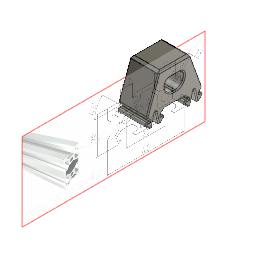
ENDER3_RUBBER_FEET_v2 (Autodesk Fusion 360 design; units mm, degrees)
Autodesk Fusion 360 part; units mm, degrees
sketch "Sketch1" plane through (0, 0, 0) normal (1, 0, 0) x (0, 1, 0)
  line L0 (20, 11.6667) -> (-20, 11.6667)
  line L1 (-20, 11.6667) -> (-20, -11.6667)
  line L2 (-20, -11.6667) -> (20, -11.6667)
  line L3 (20, -11.6667) -> (20, 11.6667)
  line L4 (20, 11.6667) -> (-20, -11.6667) construction
  line L5 (-20, 11.6667) -> (20, -11.6667) construction
  line L6 (-15.4, 8.6) -> (-15.4, 10.1)
  line L7 (-15.4, 10.1) -> (-13.2, 10.2)
  line L8 (-13.2, 10.2) -> (-13.2, 10.4)
  line L9 (-13.2, 10.4) -> (-14.6998, 11.8912)
  line L10 (-15.4, 8.6) -> (-12.8, 6.1)
  line L11 (-12.8, 6.1) -> (-7.2, 6.1)
  line L12 (-7.2, 6.1) -> (-4.6, 8.6)
  line L13 (-4.6, 8.6) -> (-4.6, 10)
  line L14 (-4.6, 10) -> (-6.9, 10)
  line L15 (-6.9, 10) -> (-6.9, 10.4)
  line L16 (-6.9, 10.4) -> (-5.2, 11.9)
  line L17 (-5.2, 11.9) -> (5.1942, 11.9)
  line L18 (5.1942, 11.9) -> (6.9277, 10.3512)
  line L19 (6.9277, 10.3512) -> (6.9277, 10.1)
  line L20 (6.9277, 10.1) -> (4.6, 10.1)
  line L21 (4.6, 10.1) -> (4.6, 8.6)
  line L22 (4.6, 8.6) -> (7.1681, 6.1554)
  line L23 (7.1681, 6.1554) -> (12.8, 6.1554)
  line L24 (12.8, 6.1554) -> (15.4, 8.6)
  line L25 (15.4, 8.6) -> (15.4, 10.1)
  line L26 (15.4, 10.1) -> (13.1, 10.1)
  line L27 (13.1, 10.1) -> (13.1, 10.4)
  line L28 (13.1, 10.4) -> (14.7, 11.9)
  line L29 (-12.95, 10.504) -> (-14.5235, 12.0685)
  line L30 (-12.95, 9.9611) -> (-12.95, 10.504)
  line L31 (-15.15, 9.8611) -> (-12.95, 9.9611)
  line L32 (-15.15, 8.7064) -> (-15.15, 9.8611)
  line L33 (-15.15, 8.7064) -> (-12.6993, 6.35)
  line L34 (-12.6993, 6.35) -> (-7.3007, 6.35)
  line L35 (-7.3007, 6.35) -> (-4.85, 8.7064)
  line L36 (-4.85, 8.7064) -> (-4.85, 9.75)
  line L37 (-4.85, 9.75) -> (-7.15, 9.75)
  line L38 (-7.15, 9.75) -> (-7.15, 10.5128)
  line L39 (-7.15, 10.5128) -> (-5.2945, 12.15)
  line L40 (-5.2945, 12.15) -> (5.2897, 12.15)
  line L41 (5.2897, 12.15) -> (7.1777, 10.4631)
  line L42 (7.1777, 10.4631) -> (7.1777, 9.85)
  line L43 (7.1777, 9.85) -> (4.85, 9.85)
  line L44 (4.85, 9.85) -> (4.85, 8.7072)
  line L45 (4.85, 8.7072) -> (7.268, 6.4054)
  line L46 (7.268, 6.4054) -> (12.7009, 6.4054)
  line L47 (12.7009, 6.4054) -> (15.15, 8.7081)
  line L48 (15.15, 8.7081) -> (15.15, 9.85)
  line L49 (15.15, 9.85) -> (12.85, 9.85)
  line L50 (12.85, 9.85) -> (12.85, 10.5083)
  line L51 (12.85, 10.5083) -> (14.529, 12.0824)
  line L52 (-0.0024, 12.15) -> (-0.0024, 30)
  line L53 (-0.0024, 30) -> (-8, 30)
  line L54 (-8, 30) -> (-14.5235, 12.0685)
  line L55 (-0.0024, 30) -> (7.9951, 30)
  line L56 (7.9951, 30) -> (14.5186, 12.0685)
  dimension "d1" = 40
  dimension "d2" = 0.25
  measures "d1" distance of L0.start L0.end
extrude "Extrude1" add sketch "Sketch1" along normal blind 15 contours L0 L41 L42 L43 L44 L45 L46 L47 L48 L49 L50 L51 | L0 L40 L41 L51 L52 L55 L56 | L0 L29 L39 L40 L52 L53 L54 | L0 L29 L30 L31 L32 L33 L34 L35 L36 L37 L38 L39
sketch "Sketch2" plane through (15, 0, 0) normal (1, 0, 0) x (0, 1, 0)
  line L0 (7.9951, 30) -> (-8, 30)
  line L1 (-8, 30) -> (-14.5235, 12.0685)
  line L2 (-14.5235, 12.0685) -> (-12.95, 10.504)
  line L3 (-12.95, 10.504) -> (-12.95, 9.9611)
  line L4 (-12.95, 9.9611) -> (-15.15, 9.8611)
  line L5 (-15.15, 9.8611) -> (-15.15, 8.7064)
  line L6 (-15.15, 8.7064) -> (-12.6993, 6.35)
  line L7 (-12.6993, 6.35) -> (-7.3007, 6.35)
  line L8 (-7.3007, 6.35) -> (-4.85, 8.7064)
  line L9 (-4.85, 8.7064) -> (-4.85, 9.75)
  line L10 (-4.85, 9.75) -> (-7.15, 9.75)
  line L11 (-7.15, 9.75) -> (-7.15, 10.5128)
  line L12 (-7.15, 10.5128) -> (-5.2945, 12.15)
  line L13 (-5.2945, 12.15) -> (5.2897, 12.15)
  line L14 (5.2897, 12.15) -> (7.1777, 10.4631)
  line L15 (7.1777, 10.4631) -> (7.1777, 9.85)
  line L16 (7.1777, 9.85) -> (4.85, 9.85)
  line L17 (4.85, 9.85) -> (4.85, 8.7072)
  line L18 (4.85, 8.7072) -> (7.268, 6.4054)
  line L19 (7.268, 6.4054) -> (12.7009, 6.4054)
  line L20 (12.7009, 6.4054) -> (15.15, 8.7081)
  line L21 (15.15, 8.7081) -> (15.15, 9.85)
  line L22 (15.15, 9.85) -> (12.85, 9.85)
  line L23 (12.85, 9.85) -> (12.85, 10.5083)
  line L24 (12.85, 10.5083) -> (14.5175, 12.0716)
  line L25 (14.5175, 12.0716) -> (7.9951, 30)
  line L26 (-10, 6.35) -> (-10, 13.85)
  line L27 (-10, 13.85) -> (-11.75, 6.35)
  line L28 (-11.75, 6.35) -> (-10, 6.35)
  line L29 (-0.0024, 30) -> (-0.0024, 12.15)
  line L30 (-10, 13.85) -> (-8.25, 6.35)
  line L31 (-8.25, 6.35) -> (-10, 6.35)
  line L32 (11.7451, 6.35) -> (9.9951, 6.35)
  line L33 (9.9951, 13.85) -> (11.7451, 6.35)
  line L34 (9.9951, 13.85) -> (8.2451, 6.35)
  line L35 (8.2451, 6.35) -> (9.9951, 6.35)
  line L36 (-6.9973, 17.4) -> (6.9924, 17.4)
  line L37 (6.9924, 17.4) -> (4.3185, 24.75)
  line L38 (4.3185, 24.75) -> (-4.3233, 24.75)
  line L39 (-4.3233, 24.75) -> (-6.9973, 17.4)
  dimension "d5" = 1.75
  dimension "d6" = 7.5
  dimension "d7" = 5.25
  measures "d5" distance of L26.start L27.end
  measures "d6" distance of L26.start L26.end
extrude "Extrude2" cut sketch "Sketch2" against normal through all contours L29 L36 L37 L38 | L29 L36 L38 L39 | L19 L33 L34 | L7 L26 L27 L28 | L7 L26 L30 L31
fillet "Fillet1" radius 4.5 2 edges at (7.5, 6.9924, 17.4) (7.5, -6.9973, 17.4)
fillet "Fillet2" radius 2.5 2 edges at (7.5, 4.3185, 24.75) (7.5, -4.3233, 24.75)
fillet "Fillet3" radius 1 14 edges at (7.5, 15.15, 9.85) (7.5, 15.15, 8.7081) (7.5, 4.85, 9.85) (7.5, 4.85, 8.7072) (7.5, 12.7009, 6.4054) (7.5, 7.268, 6.4054) (7.5, -4.85, 9.75) (7.5, -4.85, 8.7064) (7.5, -7.3007, 6.35) (7.5, -12.6993, 6.35) (7.5, -15.15, 8.7064) (7.5, -15.15, 9.8611) (7.5, -14.5235, 12.0685) (7.5, 14.5175, 12.0716)
fillet "Fillet4" radius 0.25 2 edges at (7.5, 9.9951, 13.85) (7.5, -10, 13.85)
chamfer "Chamfer1" distance 1 angle 45 4 edges at (7.5, -8, 30) (0, -0.0024, 30) (7.5, 7.9951, 30) (15, -0.0024, 30)
chamfer "Chamfer2" distance 0.5 angle 45 12 edges at (0, 4.0159, 19.0098) (0, -0.0024, 17.4) (0, -4.0208, 19.0098) (0, -4.1464, 24.1662) (0, -0.0024, 24.75) (0, 4.1415, 24.1662) (15, -4.1464, 24.1662) (15, -4.0208, 19.0098) (15, -0.0024, 17.4) (15, 4.0159, 19.0098) (15, 4.1415, 24.1662) (15, -0.0024, 24.75)
chamfer "Chamfer3" distance 0.5 angle 45 78 edges at (15, -11.3344, 20.8345) (15, -14.3413, 12.1092) (15, -13.5102, 11.061) (15, -12.95, 10.2325) (15, -13.4602, 9.9379) (15, -14.8608, 9.2682) (15, -13.8038, 7.412) (15, -12.6701, 6.4224) (15, -12.0233, 6.35) (15, -10.9967, 9.5783) (15, -10, 12.9998) (15, -9.0033, 9.5783) (15, -7.9767, 6.35) (15, -7.3299, 6.4224) (15, -6.2824, 7.3292) (15, -5.3199, 9.1236) (15, -6.6987, 9.75) (15, -7.15, 10.1314) (15, -6.2223, 11.3314) (15, -0.0024, 12.15) (15, 6.2337, 11.3065) (15, 7.1777, 10.1565) (15, 6.664, 9.85) (15, 5.2218, 9.2213) (15, 6.2196, 7.4034) (15, 7.2966, 6.4768) (15, 7.963, 6.4054) (15, 9.0049, 9.606) (15, 9.9951, 12.9998) (15, 10.9854, 9.606) (15, 13.3455, 9.85) (15, 14.7707, 9.2184) (15, 13.7579, 7.3991) (15, 12.6731, 6.4757) (15, 12.0184, 6.4054) (15, 12.85, 10.1792) (15, 13.443, 11.0643) (15, 14.3248, 12.1176) (15, 11.3254, 20.8458) (0, -11.3344, 20.8345) (0, -14.3413, 12.1092) (0, -13.5102, 11.061) (0, -12.95, 10.2325) (0, -13.4602, 9.9379) (0, -14.8608, 9.2682) (0, -13.8038, 7.412) (0, -12.6701, 6.4224) (0, -12.0233, 6.35) (0, -9.0033, 9.5783) (0, -10, 12.9998) (0, -10.9967, 9.5783) (0, -7.9767, 6.35) (0, -7.3299, 6.4224) (0, -6.2824, 7.3292) (0, -5.3199, 9.1236) (0, -6.6987, 9.75) (0, -7.15, 10.1314) (0, -6.2223, 11.3314) (0, -0.0024, 12.15) (0, 6.2337, 11.3065) (0, 7.1777, 10.1565) (0, 6.664, 9.85) (0, 5.2218, 9.2213) (0, 6.2196, 7.4034) (0, 7.2966, 6.4768) (0, 7.963, 6.4054) (0, 10.9854, 9.606) (0, 9.9951, 12.9998) (0, 9.0049, 9.606) (0, 12.0184, 6.4054) (0, 12.6731, 6.4757) (0, 13.7579, 7.3991) (0, 14.7707, 9.2184) (0, 13.3455, 9.85) (0, 12.85, 10.1792) (0, 13.443, 11.0643) (0, 14.3248, 12.1176) (0, 11.3254, 20.8458)
